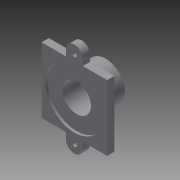
# Autodesk Inventor part: CameraLensThread
Saved by Autodesk Inventor 2015 (Build 190159000, 159)
## iProperties
Created: 2015-03-20
Part Number: CameraLensThread
Material: Generic
Document SubType Name: Modeling
Designer: Akovo_000
Density: 1 g/cm^3
Appearance: Default
Author: Akovo_000
Autodesk Inventor part; units mm, degrees
ref_plane "YZ Plane" through (0, 0, 0) normal (1, 0, 0) x (0, 1, 0)
ref_plane "XZ Plane" through (0, 0, 0) normal (0, 1, 0) x (-1, 0, 0)
ref_plane "XY Plane" through (0, 0, 0) normal (0, 0, 1) x (1, 0, 0)
sketch "Sketch1" plane through (0, 0, 0) normal (0, 1, 0) x (-1, 0, 0)
  line L0 (12.3821, 18.3008) -> (-14.8179, 18.3008)
  line L1 (-14.8179, 18.3008) -> (-14.8179, -8.8992)
  line L2 (-14.8179, -8.8992) -> (12.3821, -8.8992)
  line L3 (12.3821, -8.8992) -> (12.3821, 18.3008)
  line L4 (12.3821, -8.8992) -> (-14.8179, -8.8992)
  line L5 (-1.2179, 18.3008) -> (2.2821, 18.3008)
  line L6 (2.2821, 18.3008) -> (2.2821, 20.8008)
  line L7 (-1.2179, 18.3008) -> (-4.7179, 18.3008)
  line L8 (-4.7179, 18.3008) -> (-4.7179, 20.8008)
  arc A0 (2.2821, 20.8008) -> (-4.7179, 20.8008) centre (-1.2179, 20.8008) ccw
  line L9 (-1.2179, -8.8992) -> (-4.7179, -8.8992)
  line L10 (-4.7179, -8.8992) -> (-4.7179, -11.3992)
  line L11 (-1.2179, -8.8992) -> (2.2821, -8.8992)
  line L12 (2.2821, -8.8992) -> (2.2821, -11.3992)
  arc A1 (-4.7179, -11.3992) -> (2.2821, -11.3992) centre (-1.2179, -11.3992) ccw
  circle A2 centre (-1.2179, 20.8008) radius 1.05
  circle A3 centre (-1.2179, -11.3992) radius 1.05
  circle A4 centre (-1.2179, 4.7008) radius 12.05
  circle A5 centre (-1.2179, 4.7008) radius 5.91
  point P0 (0, 0)
  point P1 (12.0321, 4.7008)
  point P2 (-14.4679, 4.7008)
  dimension "d4" = 27.2
  dimension "d5" = 27.2
  dimension "d10" = 2.5
  dimension "d11" = 3.5
  dimension "d12" = 2.5
  dimension "d13" = 3.5
  dimension "d14" = 2.1
  dimension "d15" = 2.1
  dimension "d16" = 24.1
  dimension "d17" = 11.82
  constraints: 26 end point, 6 centre point, 5 horizontal, 5 perpendicular, 4 point on circle, 3 coincident, 2 midpoint, 2 parallel
  measures "d4" distance of L3.start L1.end
  measures "d5" distance of L1.end L1.start
  measures "d10" distance of L6.end L5.end
  measures "d11" radius of A0
  measures "d12" distance of L10.end L9.end
  measures "d13" radius of A1
  measures "d14" diameter of A2
  measures "d15" diameter of A3
  measures "d16" diameter of A4
  measures "d17" diameter of A5
extrude "Extrusion1" add sketch "Sketch1" along normal blind 1 contours L3 L2 L1 L0 | L0 L8 A0 L6 | L12 A1 L10 L2
sketch "Sketch2" plane through (0, 1, 0) normal (0, 1, 0) x (1, 0, 0)
  line L0 (14.8179, -18.3008) -> (14.8179, 8.8992)
  line L1 (-12.3821, 8.8992) -> (-12.3821, -18.3008)
  circle A0 centre (1.2179, -4.7008) radius 5.91
  circle A1 centre (1.2179, -4.7008) radius 7.5
  line L2 (-12.3821, -18.3008) -> (14.8179, -18.3008)
  line L3 (14.8179, -18.3008) -> (-12.3821, -18.3008)
  line L4 (14.8179, 8.8992) -> (-12.3821, 8.8992)
  line L5 (1.2179, 8.8992) -> (4.7179, 8.8992)
  line L6 (-2.2821, 8.8992) -> (-2.2821, 11.3992)
  line L7 (4.7179, 8.8992) -> (4.7179, 11.3992)
  circle A2 centre (1.2179, 11.3992) radius 1.05
  arc A3 (4.7179, 11.3992) -> (-2.2821, 11.3992) centre (1.2179, 11.3992) ccw
  line L8 (1.2179, 8.8992) -> (-2.2821, 8.8992)
  line L9 (1.2179, -18.3008) -> (-2.2821, -18.3008)
  line L10 (1.2179, -18.3008) -> (4.7179, -18.3008)
  line L11 (4.7179, -18.3008) -> (4.7179, -20.8008)
  circle A4 centre (1.2179, -20.8008) radius 1.05
  arc A5 (-2.2821, -20.8008) -> (4.7179, -20.8008) centre (1.2179, -20.8008) ccw
  line L12 (-2.2821, -18.3008) -> (-2.2821, -20.8008)
  point P0 (0, 0)
  point P1 (14.4679, -4.7008)
  point P2 (-12.0321, -4.7008)
  dimension "d20" = 27.2
  dimension "d21" = 27.2
  dimension "d22" = 2.5
  dimension "d23" = 3.5
  dimension "d24" = 2.5
  dimension "d25" = 3.5
  dimension "d26" = 2.1
  dimension "d27" = 2.1
  dimension "d28" = 15
  dimension "d29" = 11.82
  constraints: 26 end point, 6 centre point, 5 horizontal, 5 perpendicular, 4 point on circle, 3 coincident, 2 midpoint, 2 parallel
  measures "d20" distance of L0.start L1.end
  measures "d21" distance of L1.end L1.start
  measures "d22" distance of L7.end L5.end
  measures "d23" radius of A3
  measures "d24" distance of L12.end L9.end
  measures "d25" radius of A5
  measures "d26" diameter of A2
  measures "d27" diameter of A4
  measures "d28" diameter of A1
  measures "d29" diameter of A0
extrude "Extrusion2" add sketch "Sketch2" along normal blind 2 contours L2 L1 L4 L0 | L11 A5 L12 L2 | L4 L6 A3 L7 | A1
sketch "Sketch3" plane through (0, 3, 0) normal (0, 1, 0) x (1, 0, 0)
  circle A0 centre (1.2179, -4.7008) radius 5.91
  circle A1 centre (1.2179, -4.7008) radius 8
  point P0 (0, 0)
  point P1 (0, 0)
  dimension "d40" = 16
  dimension "d41" = 11.82
  constraints: 2 centre point, 1 coincident
  measures "d40" diameter of A1
  measures "d41" diameter of A0
extrude "Extrusion3" add sketch "Sketch3" along normal blind 10
body "Solid1"
